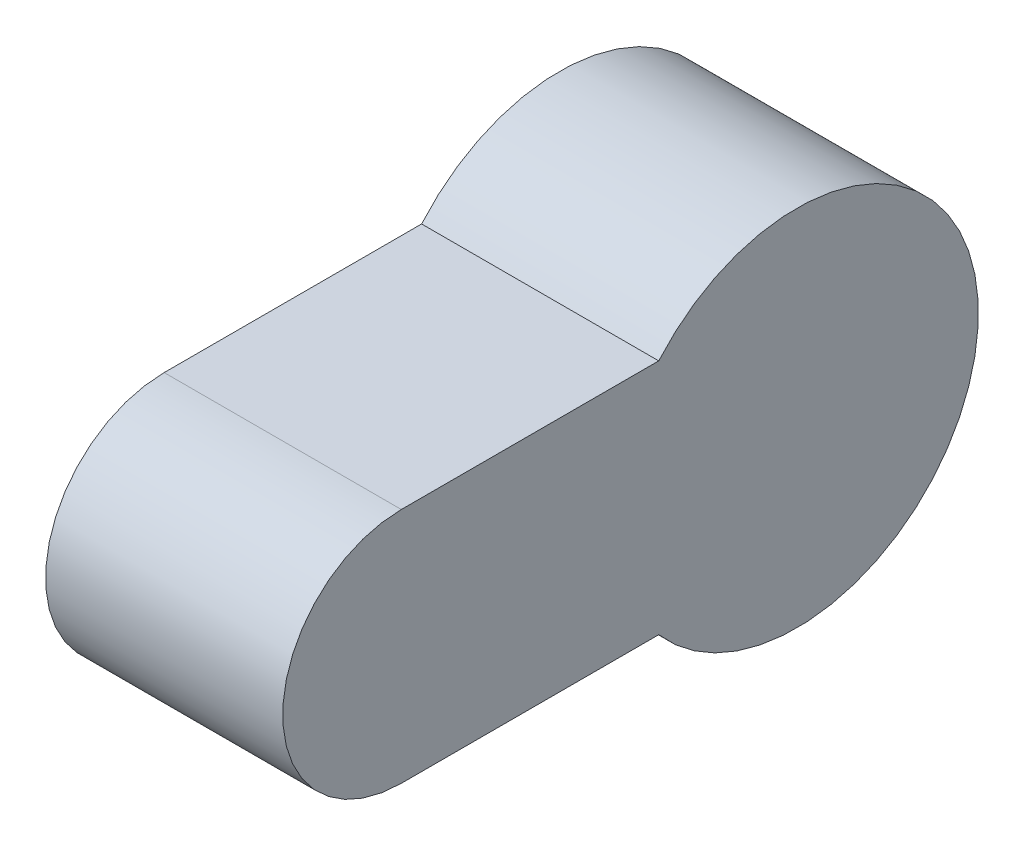
# Autodesk Inventor part: hip_back
Saved by Autodesk Inventor 2020.2 (Build 242310000, 310)
## iProperties
Created: 2021-09-18
Part Number: hip_back
Material: Generic
Document SubType Name: Modeling
Designer: boxi
Density: 1 g/cm^3
Appearance: Clear - Blue
Author: boxi
Autodesk Inventor part; units mm, degrees
ref_plane "YZ Plane" through (0, 0, 0) normal (1, 0, 0) x (0, 1, 0)
ref_plane "XZ Plane" through (0, 0, 0) normal (0, 1, 0) x (-1, 0, 0)
ref_plane "XY Plane" through (0, 0, 0) normal (0, 0, 1) x (1, 0, 0)
sketch "Sketch1" plane through (0, 0, 0) normal (1, 0, 0) x (0, 1, 0)
  circle A0 centre (0, 0) radius 30
  circle A1 centre (0, -100) radius 46
  line L0 (-64.4, 0) -> (64.4, 0) construction
  line L1 (0, -181.2) -> (0, 65.2) construction
  line L2 (30, 0) -> (30, -65.1288)
  line L3 (-30, 0) -> (-30, -65.1288)
  circle A2 centre (0, 0) radius 15
  dimension "d0" = 60
  dimension "d1" = 92
  dimension "d2" = 60
  dimension "d3" = 100
  dimension "d12" = 30
  constraints: 4 end point, 4 point on circle, 3 centre point, 2 coincident, 2 parallel, 1 point on line, 1 other
  measures "d0" diameter of A0
  measures "d1" diameter of A1
  measures "d2" distance between parallel lines of L2 L3
  measures "d3" distance from line of A1.centre L0
  measures "d12" diameter of A2
extrude "Extrusion1" add sketch "Sketch1" along normal blind 60 contours A0 | L2 A1 L3 A0 | A1 | A2
equation "\"d0\" = d2"
body "Solid1"
